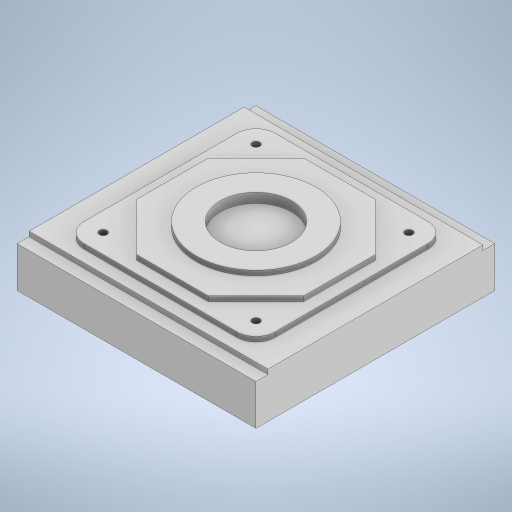
# Autodesk Inventor part: A2P3
Saved by Autodesk Inventor 2023.2 (Build 272271000, 271)
## iProperties
Created: 2023-01-23
Part Number: A2P3
Material: Generic
Document SubType Name: Modeling
Designer: manas
Density: 1 g/cm^3
Appearance: Default
Author: manas
Autodesk Inventor part; units mm, degrees
ref_plane "YZ Plane" through (0, 0, 0) normal (1, 0, 0) x (0, 1, 0)
ref_plane "XZ Plane" through (0, 0, 0) normal (0, 1, 0) x (-1, 0, 0)
ref_plane "XY Plane" through (0, 0, 0) normal (0, 0, 1) x (1, 0, 0)
sketch "Sketch1" plane through (0, 0, 0) normal (0, 1, 0) x (-1, 0, 0)
  line L0 (50, 50) -> (-50, 50)
  line L1 (-50, 50) -> (-50, -50)
  line L2 (-50, -50) -> (50, -50)
  line L3 (50, -50) -> (50, 50)
  line L4 (50, 50) -> (-50, -50) construction
  line L5 (-50, 50) -> (50, -50) construction
  point P0 (0, 0)
  dimension "d0" = 100
  dimension "d1" = 100
  constraints: 12 end point, 2 midpoint, 2 parallel, 1 horizontal, 1 perpendicular
  measures "d0" distance of L2.end L1.end
  measures "d1" distance of L1.end L0.end
extrude "Extrusion1" add sketch "Sketch1" along normal blind 17
sketch "Sketch2" plane through (0, 17, 0) normal (0, 1, 0) x (1, 0, 0)
  line L0 (-50, 50) -> (-50, -50) projected
  line L1 (50, -50) -> (50, 50) projected
  line L2 (-50, -45) -> (50, -45)
  line L3 (-50, -50) -> (50, -50) projected
  line L4 (-50, 45) -> (50, 45)
  line L5 (50, 50) -> (-50, 50) projected
  point P0 (0, 0)
  dimension "d4" = 5
  dimension "d5" = 5
  constraints: 4 end point, 4 point on line, 2 horizontal
  measures "d4" distance between parallel lines of L3 L2
  measures "d5" distance between parallel lines of L5 L4
extrude "Extrusion2" add sketch "Sketch2" along normal blind 2 contours L4 L1 L2 L0
sketch "Sketch3" plane through (0, 19, 0) normal (0, 1, 0) x (1, 0, 0)
  line L0 (-32, -40) -> (32, -40)
  line L1 (40, -32) -> (40, 32)
  line L2 (32, 40) -> (-32, 40)
  line L3 (-40, 32) -> (-40, -32)
  line L4 (-40, -40) -> (40, 40) construction
  line L5 (40, -40) -> (-40, 40) construction
  arc A0 (32, -40) -> (40, -32) centre (32, -32) ccw
  arc A1 (40, 32) -> (32, 40) centre (32, 32) ccw
  arc A2 (-32, 40) -> (-40, 32) centre (-32, 32) ccw
  arc A3 (-40, -32) -> (-32, -40) centre (-32, -32) ccw
  point P0 (0, 0)
  dimension "d8" = 80
  dimension "d9" = 80
  dimension "d10" = 8
  constraints: 12 end point, 8 point on circle, 8 point on line, 8 tangent, 4 centre point, 3 equal radius, 2 midpoint, 2 parallel, 1 horizontal, 1 perpendicular
  measures "d8" distance of L5.end L4.end
  measures "d9" distance of L4.end L5.start
  measures "d10" radius of A0
extrude "Extrusion3" add sketch "Sketch3" along normal blind 2
sketch "Sketch4" plane through (0, 21, 0) normal (0, 1, 0) x (1, 0, 0)
  line L0 (35, -15) -> (35, 15)
  line L1 (-35, 15) -> (-35, -15)
  line L2 (-35, -15) -> (35, 15) construction
  line L3 (35, -15) -> (-35, 15) construction
  line L4 (50, -45) -> (50, 45) projected
  line L5 (-50, -50) -> (50, -50) projected
  line L6 (-15, -35) -> (15, -35)
  line L7 (15, 35) -> (-15, 35)
  line L8 (-15, -35) -> (15, 35) construction
  line L9 (15, -35) -> (-15, 35) construction
  line L10 (-15, -35) -> (-35, -15)
  line L11 (-35, 15) -> (-15, 35)
  line L12 (15, 35) -> (35, 15)
  line L13 (15, -35) -> (35, -15)
  point P0 (0, 0)
  dimension "d13" = 85
  dimension "d16" = 85
  constraints: 24 end point, 4 midpoint, 2 parallel, 1 horizontal
  measures "d13" distance between parallel lines of L4 L1
  measures "d16" distance between parallel lines of L5 L7
extrude "Extrusion4" add sketch "Sketch4" along normal blind 2
sketch "Sketch5" plane through (0, 23, 0) normal (0, 1, 0) x (1, 0, 0)
  circle A0 centre (0, 0) radius 25
  dimension "d19" = 50
  constraints: 1 centre point, 1 coincident
  measures "d19" diameter of A0
extrude "Extrusion5" add sketch "Sketch5" along normal blind 2
sketch "Sketch6" plane through (0, 25, 0) normal (0, 1, 0) x (1, 0, 0)
  circle A0 centre (0, 0) radius 15
  dimension "d22" = 30
  constraints: 1 centre point, 1 coincident
  measures "d22" diameter of A0
extrude "Extrusion6" cut sketch "Sketch6" against normal blind 4
sketch "Sketch7" plane through (0, 21, 0) normal (0, 1, 0) x (1, 0, 0)
  circle A0 centre (-32, -32) radius 1.5
  line L0 (-50, -50) -> (50, -50) projected
  line L1 (-50, 45) -> (-50, -45) projected
  circle A1 centre (-32, 32) radius 1.5
  circle A2 centre (32, -32) radius 1.5
  circle A3 centre (32, 32) radius 1.5
  point P0 (0, 0)
  dimension "d25" = 3
  dimension "d26" = 18
  dimension "d27" = 18
  dimension "d30" = 64
  dimension "d33" = 64
  constraints: 4 centre point, 1 horizontal, 1 vertical, 6 other
  measures "d25" diameter of A0
  measures "d26" distance from line of L0 A0.centre
  measures "d27" distance from line of L1 A0.centre
  measures "d30" distance of A0.centre A1.centre
  measures "d33" distance of A0.centre A2.centre
hole "Hole2" at (-32, 21, 32) at (-32, 21, -32) at (32, 21, -32) at (32, 21, 32) direction (0, -1, 0) diameter 3.1211 depth 9.1 tip angle 118 thread size "M3.5x0.35" class "6H" standard "ANSI Metric M Profile"
body "Solid1"
